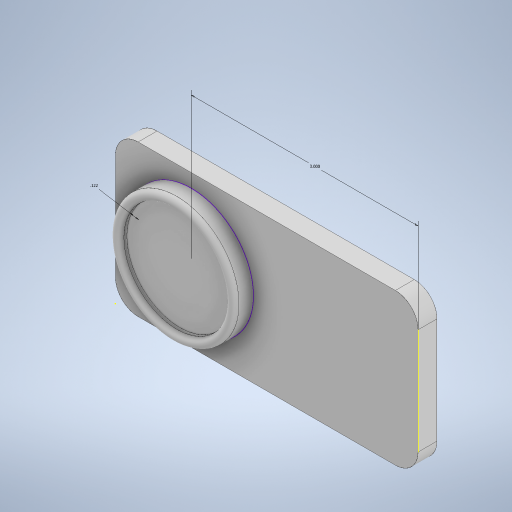
# Autodesk Inventor part: Control Panel
Saved by Autodesk Inventor 2023.2 (Build 272271030, 271C)
## iProperties
Created: 2023-02-27
Part Number: Control Panel
Material: Generic
Document SubType Name: Modeling
Designer: abhim
Density: 1 g/cm^3
Appearance: Default
Author: abhim
Autodesk Inventor part; units mm, degrees
ref_plane "YZ Plane" through (0, 0, 0) normal (1, 0, 0) x (0, 1, 0)
ref_plane "XZ Plane" through (0, 0, 0) normal (0, 1, 0) x (-1, 0, 0)
ref_plane "XY Plane" through (0, 0, 0) normal (0, 0, 1) x (1, 0, 0)
sketch "Sketch1" plane through (0, 0, 0) normal (0, 0, 1) x (1, 0, 0)
  line L0 (0, 0) -> (101.6, 0)
  line L1 (101.6, 0) -> (101.6, 50.8)
  line L2 (101.6, 50.8) -> (0, 50.8)
  line L3 (0, 50.8) -> (0, 0)
  dimension "d0" = 101.6
  dimension "d1" = 50.8
  constraints: 8 end point, 2 parallel, 1 horizontal, 1 perpendicular
  measures "d0" distance of L2.end L1.end
  measures "d1" distance of L1.end L0.end
extrude "Extrusion1" add sketch "Sketch1" along normal blind 6.35
fillet "Fillet1" radius 7.62 4 edges at (101.6, 50.8, 3.175) (101.6, 0, 3.175) (0, 50.8, 3.175) (0, 0, 3.175)
sketch "Sketch2" plane through (0, 0, 6.35) normal (0, 0, 1) x (1, 0, 0)
  circle A0 centre (25.4, 25.4) radius 20.8748
  line L0 (101.6, 7.62) -> (101.6, 43.18) projected
  circle A1 centre (25.4, 25.4) radius 17.78
  point P0 (0, 0)
  dimension "d5" = 76.2
  dimension "d13" = 3.0948
  constraints: 2 centre point, 1 coincident
  measures "d5" distance from line of L0 A0.centre
  measures "d13" radial gap between concentric circles of A0 A1
extrude "Extrusion2" add sketch "Sketch2" along normal blind 6.35 contours A0 | A1
extrude "Extrusion3" cut sketch "Sketch2" along normal blind 6.35 contours A1
extrude "Extrusion4" add sketch "Sketch2" along normal blind 3.81 contours A1
fillet "Fillet3" radius 1.5474 2 edges at (4.5252, 25.4, 12.7) (7.62, 25.4, 12.7)
body "Solid1"
